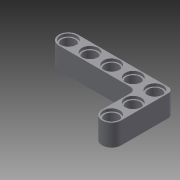
# Autodesk Inventor part: technic L 5 barrenos
Saved by Autodesk Inventor 2013 (Build 170138000, 138)
## iProperties
Created: 2013-04-04
Part Number: technic L 5 barrenos
Material: Generic
Document SubType Name: Modeling
Designer: Davila
Density: 1 g/cm^3
Author: Davila
Autodesk Inventor part; units mm, degrees
ref_plane "YZ Plane" through (0, 0, 0) normal (1, 0, 0) x (0, 1, 0)
ref_plane "XZ Plane" through (0, 0, 0) normal (0, 1, 0) x (-1, 0, 0)
ref_plane "XY Plane" through (0, 0, 0) normal (0, 0, 1) x (1, 0, 0)
sketch "Sketch1" plane through (0, 0, 0) normal (0, 0, 1) x (1, 0, 0)
  arc A0 (0, 0) -> (0, -7) centre (0, -3.5) ccw
  circle A1 centre (0, -3.5) radius 2.5
  circle A2 centre (0, -3.5) radius 3
  circle A3 centre (32, -3.5) radius 2.5
  circle A4 centre (32, -3.5) radius 3
  circle A5 centre (8, -3.5) radius 2.5
  circle A6 centre (8, -3.5) radius 3
  circle A7 centre (16, -3.5) radius 3
  circle A8 centre (16, -3.5) radius 2.5
  circle A9 centre (24, -3.5) radius 3
  circle A10 centre (24, -3.5) radius 2.5
  circle A11 centre (32, -19.5) radius 3
  circle A12 centre (32, -19.5) radius 2.5
  line L0 (28.5, -19.5) -> (28.5, -7)
  line L1 (35.5, -19.5) -> (35.5, -7)
  circle A13 centre (32, -11.5) radius 2.5
  circle A14 centre (32, -11.5) radius 3
  arc A15 (28.5, -19.5) -> (35.5, -19.5) centre (32, -19.5) ccw
  line L2 (35.5, -7) -> (35.5, 0)
  line L3 (0, -7) -> (28.5, -7)
  line L4 (0, 0) -> (35.5, 0)
  constraints: 16 centre point, 10 end point, 8 coincident, 4 point on circle, 2 parallel, 2 tangent, 1 perpendicular
extrude "Extrusion1" add sketch "Sketch1" along normal blind 8 contours L4 L2 L1 A15 L0 L3 A0 | A2 | A4 | A6 | A7 | A9 | A11 | A14
extrude "Extrusion2" cut sketch "Sketch1" along normal blind 1 contours A2 | A4 | A6 | A7 | A9 | A11 | A14
sketch "Sketch2" plane through (0, 0, 8) normal (0, 0, 1) x (1, 0, 0)
  circle A0 centre (32, -11.5) radius 2.5 projected
  circle A1 centre (32, -19.5) radius 2.5 projected
  circle A2 centre (24, -3.5) radius 2.5 projected
  circle A3 centre (16, -3.5) radius 2.5 projected
  circle A4 centre (8, -3.5) radius 2.5 projected
  circle A5 centre (32, -3.5) radius 2.5 projected
  circle A6 centre (0, -3.5) radius 2.5 projected
  circle A7 centre (0, -3.5) radius 3 projected
  circle A8 centre (8, -3.5) radius 3 projected
  circle A9 centre (16, -3.5) radius 3 projected
  circle A10 centre (24, -3.5) radius 3 projected
  circle A11 centre (32, -3.5) radius 3 projected
  circle A12 centre (32, -11.5) radius 3 projected
  circle A13 centre (32, -19.5) radius 3 projected
extrude "Extrusion3" cut sketch "Sketch2" against normal blind 1
fillet "Fillet1" radius 2 1 edges at (35.5, 0, 4)
fillet "Fillet2" radius 2 1 edges at (28.5, -7, 4)
body "Solid1"
